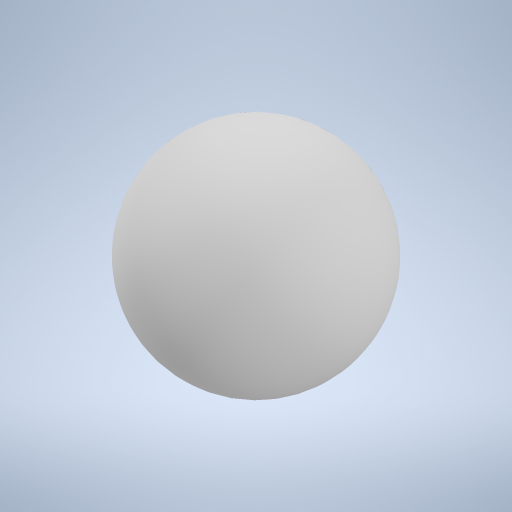
# Autodesk Inventor part: Center
Saved by Autodesk Inventor 2023 (Build 270158000, 158)
## iProperties
Created: 2022-10-18
Part Number: Center
Material: Generic
Document SubType Name: Modeling
Designer: benni
Density: 1 g/cm^3
Appearance: Default
Author: benni
Autodesk Inventor part; units mm, degrees
ref_plane "YZ Plane" through (0, 0, 0) normal (1, 0, 0) x (0, 1, 0)
ref_plane "XZ Plane" through (0, 0, 0) normal (0, 1, 0) x (-1, 0, 0)
ref_plane "XY Plane" through (0, 0, 0) normal (0, 0, 1) x (1, 0, 0)
sketch "Sketch1" plane through (0, 0, 0) normal (1, 0, 0) x (0, 1, 0)
  line L0 (0, 0) -> (2, 0)
  arc A0 (-2, 0) -> (2, 0) centre (0, 0) ccw
  line L1 (2, 0) -> (-2, 0)
  dimension "d0" = 2
  constraints: 4 end point, 2 horizontal, 2 point on circle, 1 centre point, 1 coincident
  measures "d0" distance of L0.start L0.end
revolve "Revolution1" add sketch "Sketch1" angle 360 about axis through (0, 0, 0) along (0, 1, 0)
body "Solid1"
